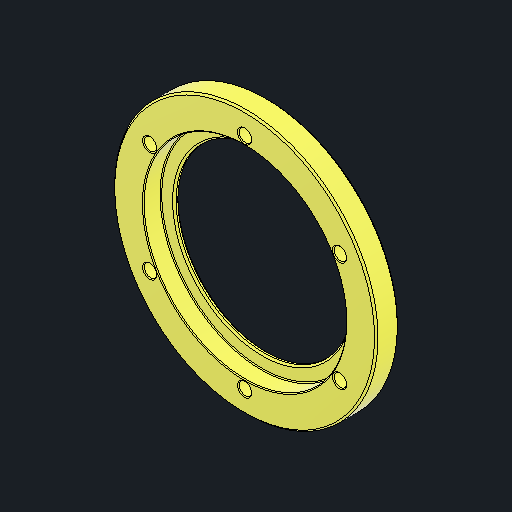
# Autodesk Inventor part: akf-100-window
Saved by Autodesk Inventor 2026 (Build 300175050, 175E)
## iProperties
Created: 2025-12-12
Part Number: akf-100-window
Material: ABS Plastic
Document SubType Name: Modeling
Designer: kuzmin
Density: 1.06 g/cm^3
Appearance: Smooth - Yellow
Author: kuzmin
Autodesk Inventor part; units mm, degrees
ref_plane "YZ Plane" through (0, 0, 0) normal (1, 0, 0) x (0, 1, 0)
ref_plane "XZ Plane" through (0, 0, 0) normal (0, 1, 0) x (-1, 0, 0)
ref_plane "XY Plane" through (0, 0, 0) normal (0, 0, 1) x (1, 0, 0)
sketch "Sketch2" plane through (0, 0, 0) normal (0, 1, 0) x (-1, 0, 0)
  line L0 (0, 0) -> (0, 13)
  line L1 (50, 0) -> (75, 0)
  line L2 (75, 0) -> (75, 13)
  line L3 (75, 13) -> (57.7, 13)
  line L4 (57.7, 13) -> (57.7, 3)
  line L5 (57.7, 3) -> (50, 3)
  line L6 (50, 3) -> (50, 0)
  dimension "d1" = 100
  dimension "d2" = 150
  dimension "d3" = 115.4
  dimension "d4" = 3
  dimension "d5" = 10
  constraints: 14 end point, 4 perpendicular, 2 horizontal alignment, 2 vertical, 1 horizontal
  measures "d1" diameter of L6 L0
  measures "d2" diameter of L2 L0
  measures "d3" diameter of L4 L0
  measures "d4" distance of L5.end L1.start
  measures "d5" distance of L3.end L4.end
revolve "Revolution1" add sketch "Sketch2" angle 360 about axis through (0, 0, 0) along (0, 0, 1)
sketch "Sketch3" plane through (0, 0, 0) normal (0, 0, -1) x (-1, 0, 0)
  circle A0 centre (0, 0) radius 62.5 construction
  point P0 (0, -62.5)
  dimension "d7" = 125
  constraints: 2 vertical alignment, 1 coincident, 2 other
hole "Hole1" at (0, -62.5, 0) direction (0, 0, 1) diameter 7 end through all
pattern_circular "Circular Pattern1" count 6 over 360 about axis through (0, 0, -10) along (0, 0, 1) of "Hole1"
chamfer "Chamfer1" distance 1 angle 45 4 edges at (75, 0, 0) (50, 0, 0) (50, 0, 3) (75, 0, 13)
chamfer "Chamfer2" distance 0.5 angle 45 12 edges at (57.1577, 33, 0) (0, 66, 0) (-57.1577, 33, 0) (-57.1577, -33, 0) (0, -66, 0) (57.1577, -33, 0) (57.1577, 33, 13) (57.1577, -33, 13) (0, -66, 13) (-57.1577, -33, 13) (-57.1577, 33, 13) (0, 66, 13)
chamfer "Chamfer3" distance 0.5 angle 45 2 edges at (57.7, 0, 13) (57.7, 0, 3)
body "Solid1"
